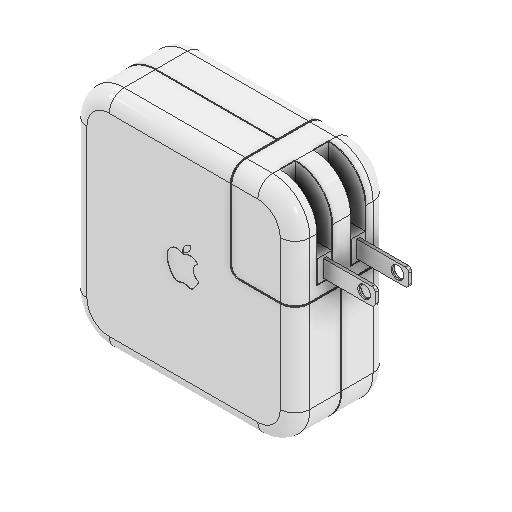
# Autodesk Inventor part: iPod Power Adapter
Saved by Autodesk Inventor 2026.2 (Build 302298000, 298)
## iProperties
Created: 2025-12-23
Part Number: iPod Power Adapter
Material: Generic
Document SubType Name: Modeling
Designer: andyeske
Density: 1 g/cm^3
Appearance: Default
Author: andyeske
Autodesk Inventor part; units mm, degrees
ref_plane "YZ Plane" through (0, 0, 0) normal (1, 0, 0) x (0, 1, 0)
ref_plane "XZ Plane" through (0, 0, 0) normal (0, 1, 0) x (-1, 0, 0)
ref_plane "XY Plane" through (0, 0, 0) normal (0, 0, 1) x (1, 0, 0)
sketch "Sketch1" plane through (0, 0, 0) normal (0, 0, 1) x (1, 0, 0)
  line L0 (-150, -150) -> (150, -150)
  line L1 (150, -150) -> (150, 150)
  line L2 (150, 150) -> (-150, 150)
  line L3 (-150, 150) -> (-150, -150)
  line L4 (-150, -150) -> (150, 150) construction
  line L5 (150, -150) -> (-150, 150) construction
  point P0 (0, 0)
  dimension "d0" = 300
  constraints: 12 end point, 2 midpoint, 2 parallel, 2 perpendicular, 1 horizontal
  measures "d0" distance of L1.end L2.end
extrude "Extrusion1" add sketch "Sketch1" along normal blind 125
fillet "Fillet1" radius 50 4 edges at (150, 150, 62.5) (-150, 150, 62.5) (150, -150, 62.5) (-150, -150, 62.5)
fillet "Fillet2" radius 20 16 edges at (0, 150, 125) (0, 150, 0) (-135.3553, 135.3553, 125) (-150, 0, 125) (-135.3553, -135.3553, 125) (0, -150, 125) (135.3553, -135.3553, 125) (150, 0, 125) (135.3553, 135.3553, 125) (-135.3553, 135.3553, 0) (-150, 0, 0) (-135.3553, -135.3553, 0) (0, -150, 0) (135.3553, -135.3553, 0) (150, 0, 0) (135.3553, 135.3553, 0)
sketch "Sketch2" plane through (0, 0, 125) normal (0, 0, 1) x (1, 0, 0)
  line L0 (100, 150) -> (-100, 150) projected
  line L1 (150, -100) -> (150, 100) projected
  line L2 (65, 150) -> (150, 150) construction
  line L3 (150, 150) -> (150, 25) construction
  line L4 (150, 25) -> (65, 25)
  line L5 (65, 25) -> (65, 150)
  line L6 (63, 150) -> (63, 23)
  line L7 (63, 23) -> (150, 23)
  line L8 (63, 150) -> (65, 150)
  point P0 (0, 0)
  dimension "d5" = 85
  dimension "d6" = 125
  dimension "d7" = 2
  dimension "d8" = 2
  constraints: 14 end point, 4 point on line, 2 parallel, 2 perpendicular, 1 collinear, 1 horizontal, 1 vertical
  measures "d5" distance of L3.end L4.end
  measures "d6" distance of L4.end L2.start
  measures "d7" distance between parallel lines of L5 L6
  measures "d8" distance between parallel lines of L7 L4
extrude "Extrusion2" cut sketch "Sketch2" against normal blind 1
sketch "Sketch3" plane through (-100, 150, 20) normal (0, 1, 0) x (1, 0, 0)
  line L0 (163, -104) -> (165, -104) projected
  line L1 (163, -104) -> (163, 0)
  line L2 (0, 0) -> (200, 0) projected
  line L3 (165, -104) -> (165, 0)
  line L4 (163, 0) -> (165, 0)
  point P0 (100, 20)
  constraints: 6 end point, 2 perpendicular, 2 point on line, 1 collinear
extrude "Extrusion3" cut sketch "Sketch3" against normal blind 1
sketch "Sketch4" plane through (150, -100, 20) normal (1, 0, 0) x (0, 0, -1)
  line L0 (-104, 125) -> (-104, 123) projected
  line L1 (-104, 125) -> (0, 125)
  line L2 (0, 200) -> (0, 0) projected
  line L3 (-104, 123) -> (0, 123)
  line L4 (0, 125) -> (0, 123)
  point P0 (20, 100)
  constraints: 6 end point, 2 point on line, 1 collinear, 1 horizontal, 1 perpendicular
extrude "Extrusion4" cut sketch "Sketch4" against normal blind 1
sketch "Sketch5" plane through (63, 23, 125) normal (1, 0, 0) x (0, 0, -1)
  arc A0 (20, 127) -> (0, 107) centre (20, 107) ccw projected
  arc A1 (20, 126) -> (1, 107) centre (20, 107) ccw
  line L0 (0, 107) -> (1, 107)
  line L1 (1, 0) -> (1, 113.245) projected
  line L2 (20, 126) -> (20, 127)
  point P0 (125, -23)
  dimension "d15" = 19
  constraints: 4 end point, 3 point on circle, 1 centre point, 1 point on line
  measures "d15" radius of A1
extrude "Extrusion5" cut sketch "Sketch5" along normal blind 2 contours L2 A1 L1 A0
sketch "Sketch6" plane through (63, 23, 125) normal (0, 1, 0) x (1, 0, 0)
  arc A0 (67, 0) -> (87, 20) centre (67, 20) ccw projected
  arc A1 (67, 1) -> (86, 20) centre (67, 20) ccw
  line L0 (86, 20) -> (87, 20)
  line L1 (86, 105) -> (86, 13.755) projected
  line L2 (73.245, 1) -> (0, 1) projected
  arc A2 (67, 0) -> (73.245, 1) centre (67, 20) ccw projected
  line L3 (67, 1) -> (67, 0)
  point P0 (-63, 125)
  dimension "d18" = 1
  constraints: 4 end point, 3 point on circle, 1 centre point, 1 perpendicular, 1 point on line
  measures "d18" radial gap between concentric circles of A0 A1
extrude "Extrusion6" cut sketch "Sketch6" along normal blind 2
sketch "Sketch7" plane through (0, 0, 0) normal (0, 0, -1) x (-1, 0, 0)
  line L0 (-63, 23) -> (-63, 130) projected
  line L1 (-130, 23) -> (-63, 23) projected
  line L2 (-65, 25) -> (-130, 25) projected
  line L3 (-65, 130) -> (-65, 25) projected
  line L4 (-65, 130) -> (-63, 130)
  line L5 (-130, 25) -> (-130, 23)
  point P0 (0, 0)
  constraints: 4 end point, 2 perpendicular
extrude "Extrusion7" cut sketch "Sketch7" against normal blind 1
sketch "Sketch8" plane through (63, 23, 125) normal (1, 0, 0) x (0, 0, -1)
  arc A0 (125, 107) -> (105, 127) centre (105, 107) ccw projected
  arc A1 (124, 107) -> (105, 126) centre (105, 107) ccw
  line L0 (105, 126) -> (105, 127)
  line L1 (125, 107) -> (124, 107) projected
  line L2 (124, 107) -> (125, 107)
  point P0 (125, -23)
  dimension "d23" = 1
  constraints: 4 end point, 2 point on circle, 1 centre point, 1 horizontal, 1 vertical
  measures "d23" radial gap between concentric circles of A0 A1
extrude "Extrusion8" cut sketch "Sketch8" along normal blind 2
sketch "Sketch9" plane through (63, 23, 125) normal (0, 1, 0) x (1, 0, 0)
  arc A0 (87, 105) -> (67, 125) centre (67, 105) ccw projected
  arc A1 (86, 105) -> (67, 124) centre (67, 105) ccw
  line L0 (67, 125) -> (67, 124) projected
  line L1 (67, 124) -> (67, 125)
  line L2 (86, 105) -> (87, 105)
  point P0 (-63, 125)
  dimension "d26" = 1
  constraints: 4 end point, 2 point on circle, 1 centre point, 1 horizontal, 1 vertical
  measures "d26" radial gap between concentric circles of A0 A1
extrude "Extrusion9" cut sketch "Sketch9" along normal blind 2
sketch "Sketch10" plane through (0, 0, 125) normal (0, 0, 1) x (1, 0, 0)
  line L0 (65, 25) -> (65, 130) projected
  line L1 (130, 25) -> (65, 25) projected
  arc A0 (65, 35) -> (75, 25) centre (75, 35) ccw
  line L2 (65, 35) -> (65, 25)
  point P0 (0, 0)
  dimension "d29" = 10
  constraints: 3 tangent, 2 end point, 2 point on circle, 2 point on line, 1 centre point, 1 collinear
  measures "d29" radius of A0
extrude "Extrusion10" cut sketch "Sketch10" against normal blind 1
sketch "Sketch11" plane through (0, 0, 125) normal (0, 0, 1) x (1, 0, 0)
  line L0 (63, 23) -> (63, 130) projected
  line L1 (63, 23) -> (130, 23) projected
  arc A0 (63, 35) -> (75, 23) centre (75, 35) ccw
  arc A1 (65, 35) -> (75, 25) centre (75, 35) ccw projected
  line L2 (63, 35) -> (63, 23)
  point P0 (0, 0)
  constraints: 3 tangent, 2 end point, 2 point on circle, 2 point on line, 1 centre point, 1 collinear, 1 concentric
extrude "Extrusion11" add sketch "Sketch11" against normal blind 1
sketch "Sketch12" plane through (0, 0, 0) normal (0, 0, -1) x (-1, 0, 0)
  arc A0 (-75, 25) -> (-65, 35) centre (-75, 35) ccw projected
  line L0 (-130, 25) -> (-65, 25) projected
  line L1 (-75, 25) -> (-65, 25)
  line L2 (-65, 25) -> (-65, 35)
  point P0 (0, 0)
  constraints: 4 end point, 1 horizontal, 1 perpendicular
extrude "Extrusion12" cut sketch "Sketch12" against normal blind 1
sketch "Sketch13" plane through (0, 0, 0) normal (0, 0, -1) x (-1, 0, 0)
  arc A0 (-75, 23) -> (-63, 35) centre (-75, 35) ccw projected
  line L0 (-63, 130) -> (-63, 23) projected
  line L1 (-63, 35) -> (-63, 23)
  line L2 (-63, 23) -> (-75, 23)
  point P0 (0, 0)
  constraints: 4 end point, 1 perpendicular, 1 tangent, 1 vertical
extrude "Extrusion13" add sketch "Sketch13" against normal blind 1
sketch "Sketch14" plane through (-100, 150, 105) normal (0, 1, 0) x (1, 0, 0)
  line L0 (163, 0) -> (163, 85) construction
  line L1 (163, 42.5) -> (0, 42.5) construction
  line L2 (0, 85) -> (0, 0) construction
  line L3 (0, 42) -> (163, 42)
  line L4 (163, 42) -> (163, 43)
  line L5 (163, 43) -> (0, 43)
  line L6 (0, 43) -> (0, 42)
  line L7 (0, 42) -> (163, 43) construction
  line L8 (163, 42) -> (0, 43) construction
  point P0 (100, 105)
  point P1 (81.5, 42.5)
  dimension "d38" = 1
  constraints: 14 end point, 5 midpoint, 2 parallel, 1 horizontal, 1 perpendicular, 1 point on line
  measures "d38" distance between parallel lines of L3 L5
extrude "Extrusion14" cut sketch "Sketch14" against normal blind 0.5
sketch "Sketch15" plane through (-150, -100, 20) normal (-1, 0, 0) x (0, 0, 1)
  line L0 (0, 200) -> (85, 200) construction
  line L1 (42.5, 200) -> (42.5, 0) construction
  line L2 (85, 0) -> (0, 0) construction
  line L3 (43, 0) -> (42, 0)
  line L4 (42, 0) -> (42, 200)
  line L5 (42, 200) -> (43, 200)
  line L6 (43, 200) -> (43, 0)
  line L7 (43, 0) -> (42, 200) construction
  line L8 (42, 0) -> (43, 200) construction
  point P0 (-20, 100)
  point P1 (42.5, 100)
  dimension "d41" = 1
  constraints: 14 end point, 5 midpoint, 2 parallel, 1 horizontal, 1 perpendicular, 1 point on line
  measures "d41" distance between parallel lines of L6 L4
extrude "Extrusion15" cut sketch "Sketch15" against normal blind 0.5
sketch "Sketch16" plane through (-100, -150, 20) normal (0, -1, 0) x (1, 0, 0)
  line L0 (200, 85) -> (200, 0) construction
  line L1 (200, 42.5) -> (0, 42.5) construction
  line L2 (0, 0) -> (0, 85) construction
  line L3 (200, 43) -> (0, 43)
  line L4 (0, 43) -> (0, 42)
  line L5 (0, 42) -> (200, 42)
  line L6 (200, 42) -> (200, 43)
  line L7 (200, 43) -> (0, 42) construction
  line L8 (0, 43) -> (200, 42) construction
  point P0 (100, -20)
  point P1 (100, 42.5)
  dimension "d44" = 1
  constraints: 14 end point, 5 midpoint, 2 parallel, 1 horizontal, 1 perpendicular, 1 point on line
  measures "d44" distance between parallel lines of L3 L5
extrude "Extrusion16" cut sketch "Sketch16" against normal blind 0.5
sketch "Sketch17" plane through (150, -100, 105) normal (1, 0, 0) x (0, 0, -1)
  line L0 (42.5, 0) -> (38.8069, 200) construction
  line L1 (42.5, 0) -> (42.5, 123) construction
  line L2 (85, 123) -> (0, 123) construction
  line L3 (0, 0) -> (42, 0) projected
  line L4 (43, 123) -> (42, 123)
  line L5 (42, 123) -> (42, 0)
  line L6 (42, 0) -> (43, 0)
  line L7 (43, 0) -> (43, 123)
  line L8 (43, 123) -> (42, 0) construction
  line L9 (42, 123) -> (43, 0) construction
  line L10 (85, 123) -> (85, 0) construction
  line L11 (85, 61.5) -> (42.5, 61.5) construction
  point P0 (105, 100)
  dimension "d47" = 1
  dimension "d53" = 42.5
  constraints: 18 end point, 5 midpoint, 2 parallel, 2 perpendicular, 1 horizontal, 1 point on line, 1 vertical
  measures "d47" distance between parallel lines of L5 L7
  measures "d53" distance of L11.start L11.end
extrude "Extrusion17" cut sketch "Sketch17" against normal blind 0.5
sketch "Sketch18" plane through (-150, -100, 63) normal (0, 0, -1) x (-1, 0, 0)
  arc A0 (0, 200) -> (-50, 250) centre (-50, 200) ccw projected
  arc A1 (-50, -50) -> (0, 0) centre (-50, 0) ccw projected
  arc A2 (-300, 0) -> (-250, -50) centre (-250, 0) ccw projected
  arc A3 (-299.5, 0) -> (-250, -49.5) centre (-250, 0) ccw
  arc A4 (-50, -49.5) -> (-0.5, 0) centre (-50, 0) ccw
  arc A5 (-0.5, 200) -> (-50, 249.5) centre (-50, 200) ccw
  line L0 (-0.5, 200) -> (0, 200)
  line L1 (-50, 250) -> (-50, 249.5) projected
  line L2 (0, 0) -> (-0.5, 0) projected
  line L3 (-50, -50) -> (-50, -49.5) projected
  line L4 (-250, -50) -> (-250, -49.5) projected
  line L5 (-300, 0) -> (-299.5, 0) projected
  point P0 (-150, 100)
  dimension "d50" = 0.5
  dimension "d51" = 0.5
  dimension "d52" = 0.5
  constraints: 6 point on circle, 5 point on line, 3 centre point, 2 end point, 1 horizontal
  measures "d50" radial gap between concentric circles of A2 A3
  measures "d51" radial gap between concentric circles of A1 A4
  measures "d52" radial gap between concentric circles of A0 A5
extrude "Extrusion18" cut sketch "Sketch18" along normal blind 1
sketch "Sketch19" plane through (0, 0, 125) normal (0, 0, 1) x (1, 0, 0)
  line L0 (-25.8842, 32.2382) -> (24.1158, 32.2382) construction
  line L1 (24.1158, 32.2382) -> (24.1158, -21.8992) construction
  line L2 (24.1158, -21.8992) -> (-25.8842, -21.8992) construction
  line L3 (-25.8842, -21.8992) -> (-25.8842, 32.2382) construction
  spline S0 degree 4 poles (-0.6067, 15.9177) (2.7295, 16.3934) (4.6914, 19.5945) (14.5472, 18.5482) (17.2027, 15.3244) (18.6949, 13.3249) knots 0 0 0 0 0 0.505773 1 1 1 1 1
  spline S1 degree 4 poles (18.6949, 13.3249) (17.4559, 12.3952) (13.095, 9.7666) (11.88, 0.5556) (16.3487, -4.4756) (18.9422, -6.1803) (20.1095, -6.4916) knots 0 0 0 0 0 0.441121 0.625892 1 1 1 1 1
  spline S2 degree 4 poles (20.1095, -6.4916) (19.0498, -10.0156) (18.7751, -10.1929) (13.7906, -17.7207) (11.0782, -19.5298) (7.8639, -20.2186) (5.3082, -19.0784) (0.7675, -17.5229) (-2.0147, -18.0206) (-6.006, -19.5989) (-9.1544, -20.4858) (-13.1462, -18.1919) (-14.7306, -15.8813) (-18.6351, -10.7741) (-19.3629, -8.5442) (-22.322, -1.3736) (-21.8645, 4.1613) (-21.7165, 10.1898) (-17.7625, 15.2877) (-10.9125, 18.9157) (-7.1098, 18.7842) (-2.3164, 15.9818) (-0.6067, 15.9177) knots 0 0 0 0 0 0.113024 0.15496 0.194895 0.233325 0.273058 0.315021 0.3576 0.399129 0.440951 0.48455 0.528381 0.575776 0.626758 0.678413 0.73359 0.787538 0.838503 0.887902 1 1 1 1 1
  arc A0 (9.5273, 30.1366) -> (-0.8842, 18.2584) centre (10.1214, 19.1138) ccw
  arc A1 (-0.8842, 18.2584) -> (9.5273, 30.1366) centre (-1.5571, 29.3502) ccw
  point P0 (0, 0)
  point P1 (3.3905, 17.2501)
  point P2 (7.0996, 18.2584)
  point P3 (12.4291, 17.7902)
  point P4 (16.3182, 15.9177)
  point P5 (16.3182, 11.4164)
  point P6 (13.5094, 6.771)
  point P7 (13.5609, 0.7964)
  point P8 (15.849, -3.3903)
  point P9 (18.4293, -5.6785)
  point P10 (18.6949, -10.1752)
  point P11 (16.3182, -13.7425)
  point P12 (12.7147, -18.1632)
  point P13 (10.6394, -19.4677)
  point P14 (8.1689, -19.863)
  point P15 (5.3425, -19.1514)
  point P16 (1.0358, -17.9357)
  point P17 (-2.1974, -18.2296)
  point P18 (-5.9382, -19.4854)
  point P19 (-9.2248, -19.8595)
  point P20 (-12.5651, -18.2562)
  point P21 (-14.8899, -15.7181)
  point P22 (-17.9783, -11.3749)
  point P23 (-19.5146, -8.2718)
  point P24 (-21.5699, -1.9875)
  point P25 (-21.9056, 4.2826)
  point P26 (-20.8879, 10.1017)
  point P27 (-17.1455, 15.106)
  point P28 (-12.3285, 17.7902)
  point P29 (-8.4965, 18.2584)
  point P30 (-4.0648, 16.9966)
  dimension "d59" = 50
  constraints: 4 point on circle, 2 centre point, 38 other
  measures "d59" distance of L1.end L2.end
extrude "Extrusion19" cut sketch "Sketch19" against normal blind 0.5
sketch "Sketch20" plane through (0, 0, 0) normal (0, 0, -1) x (-1, 0, 0)
  line L0 (-26.5297, 33.619) -> (23.4703, 33.619) construction
  line L1 (23.4703, 33.619) -> (23.4703, -20.5184) construction
  line L2 (23.4703, -20.5184) -> (-26.5297, -20.5184) construction
  line L3 (-26.5297, -20.5184) -> (-26.5297, 33.619) construction
  spline S0 degree 4 poles (-1.2521, 17.2985) (2.084, 17.7743) (4.046, 20.9753) (13.9017, 19.929) (16.5573, 16.7052) (18.0494, 14.7058) knots 0 0 0 0 0 0.505773 1 1 1 1 1
  spline S1 degree 4 poles (18.0494, 14.7058) (16.8105, 13.776) (12.4496, 11.1474) (11.2345, 1.9364) (15.7032, -3.0948) (18.2967, -4.7995) (19.464, -5.1108) knots 0 0 0 0 0 0.441121 0.625892 1 1 1 1 1
  spline S2 degree 4 poles (19.464, -5.1108) (18.4043, -8.6348) (18.1296, -8.8121) (13.1451, -16.3399) (10.4327, -18.149) (7.2184, -18.8378) (4.6628, -17.6976) (0.122, -16.1421) (-2.6601, -16.6398) (-6.6515, -18.218) (-9.7999, -19.1049) (-13.7916, -16.8111) (-15.3761, -14.5005) (-19.2806, -9.3932) (-20.0084, -7.1634) (-22.9675, 0.0072) (-22.51, 5.5421) (-22.362, 11.5706) (-18.4079, 16.6686) (-11.558, 20.2965) (-7.7553, 20.165) (-2.9619, 17.3626) (-1.2521, 17.2985) knots 0 0 0 0 0 0.113024 0.15496 0.194895 0.233325 0.273058 0.315021 0.3576 0.399129 0.440951 0.48455 0.528381 0.575776 0.626758 0.678413 0.73359 0.787538 0.838503 0.887902 1 1 1 1 1
  arc A0 (8.8818, 31.5175) -> (-1.5297, 19.6392) centre (9.476, 20.4946) ccw
  arc A1 (-1.5297, 19.6392) -> (8.8818, 31.5175) centre (-2.2026, 30.731) ccw
  point P0 (0, 0)
  point P1 (-0.6455, 1.3808)
  point P2 (2.745, 18.6309)
  point P3 (6.4541, 19.6392)
  point P4 (11.7836, 19.171)
  point P5 (15.6728, 17.2985)
  point P6 (15.6727, 12.7972)
  point P7 (12.8639, 8.1519)
  point P8 (12.9155, 2.1773)
  point P9 (15.2036, -2.0095)
  point P10 (17.7838, -4.2977)
  point P11 (18.0494, -8.7944)
  point P12 (15.6727, -12.3617)
  point P13 (12.0692, -16.7824)
  point P14 (9.9939, -18.0868)
  point P15 (7.5234, -18.4821)
  point P16 (4.6971, -17.7706)
  point P17 (0.3903, -16.5549)
  point P18 (-2.8429, -16.8488)
  point P19 (-6.5837, -18.1046)
  point P20 (-9.8703, -18.4787)
  point P21 (-13.2105, -16.8754)
  point P22 (-15.5354, -14.3372)
  point P23 (-18.6238, -9.994)
  point P24 (-20.1601, -6.891)
  point P25 (-22.2154, -0.6066)
  point P26 (-22.551, 5.6634)
  point P27 (-21.5333, 11.4825)
  point P28 (-17.791, 16.4868)
  point P29 (-12.974, 19.1711)
  point P30 (-9.142, 19.6392)
  point P31 (-4.7103, 18.3775)
  dimension "d79" = 50
  constraints: 4 point on circle, 2 centre point, 37 other
  measures "d79" distance of L1.end L3.start
extrude "Extrusion20" cut sketch "Sketch20" against normal blind 0.5
sketch "Sketch21" plane through (-150, -100, 20) normal (-1, 0, 0) x (0, 0, 1)
  line L0 (0, 0) -> (0, 200) construction
  line L1 (0, 100) -> (85, 100) construction
  line L2 (85, 0) -> (85, 123) construction
  circle A0 centre (42.5, 100) radius 30
  circle A1 centre (42.5, 100) radius 31
  point P0 (-20, 100)
  dimension "d85" = 60
  dimension "d86" = 1
  constraints: 2 centre point, 2 end point, 2 midpoint, 1 horizontal, 1 point on line
  measures "d85" diameter of A0
  measures "d86" radial gap between concentric circles of A0 A1
extrude "Extrusion21" cut sketch "Sketch21" against normal up to surface (0.5 mm away)
sketch "Sketch22" plane through (-150, 0, 62.5) normal (-1, 0, 0) x (0, 0, 1)
  point P0 (-62.5, 0)
extrude "Extrusion22" add sketch "Sketch21" against normal up to surface (0.5 mm away) contours A0
sketch "Sketch23" plane through (-150, 0, 62.5) normal (-1, 0, 0) x (0, 0, 1)
  circle A0 centre (0, 0) radius 30 construction
  line L0 (0, 30) -> (0, -30) construction
  line L1 (0.5, -100) -> (0.5, 23) construction
  line L2 (0, 0) -> (42.5, 0) construction
  line L3 (42.5, 100) -> (42.5, -100) construction
  line L4 (-10, -25) -> (10, -25)
  line L5 (10, -25) -> (10, 25)
  line L6 (10, 25) -> (-10, 25)
  line L7 (-10, 25) -> (-10, -25)
  line L8 (-10, -25) -> (10, 25) construction
  line L9 (10, -25) -> (-10, 25) construction
  point P0 (-62.5, 0)
  dimension "d91" = 42.5
  dimension "d92" = 20
  dimension "d93" = 50
  constraints: 16 end point, 4 midpoint, 3 parallel, 2 point on circle, 1 horizontal, 1 perpendicular
  measures "d91" distance of L2.start L2.end
  measures "d92" distance of L5.end L6.end
  measures "d93" distance of L4.end L5.end
extrude "Extrusion23" cut sketch "Sketch23" against normal blind 50
chamfer "Chamfer1" distance 0.5 angle 45 4 edges at (-150, 25, 62.5) (-150, 0, 52.5) (-150, 0, 72.5) (-150, -25, 62.5)
sketch "Sketch24" plane through (100, 150, 105) normal (0, 1, 0) x (1, 0, 0)
  line L0 (50, 0) -> (50, 85) projected
  line L1 (0, 43) -> (0, 85) projected
  line L2 (50, 75) -> (0, 75)
  line L3 (0, 75) -> (0, 55)
  line L4 (0, 55) -> (50, 55)
  line L5 (50, 55) -> (50, 75)
  line L6 (50, 30) -> (0, 30)
  line L7 (0, 30) -> (0, 10)
  line L8 (0, 10) -> (50, 10)
  line L9 (50, 10) -> (50, 30)
  line L10 (50, 85) -> (0, 85) projected
  line L11 (0, 0) -> (50, 0) projected
  point P0 (-100, 105)
  point P1 (0, 75)
  point P2 (50, 10)
  point P3 (50, 30)
  dimension "d99" = 10
  dimension "d100" = 10
  dimension "d101" = 20
  dimension "d102" = 20
  constraints: 16 end point, 4 parallel, 4 point on line, 2 horizontal, 2 perpendicular
  measures "d99" distance between parallel lines of L2 L10
  measures "d100" distance between parallel lines of L11 L8
  measures "d101" distance between parallel lines of L4 L2
  measures "d102" distance between parallel lines of L8 L6
extrude "Extrusion24" cut sketch "Sketch24" against normal blind 110 contours L8 L7 L6 L0 | L4 L1 L2 L0
fillet "Fillet3" radius 0.5 12 edges at (100, 150, 85) (150, 70, 75) (135.3553, 135.3553, 75) (150, 70, 95) (135.3553, 135.3553, 95) (100, 150, 40) (150, 70, 50) (135.3553, 135.3553, 50) (150, 70, 30) (135.3553, 135.3553, 30) (150, 40, 40) (150, 40, 85)
sketch "Sketch25" plane through (100, 40, 30) normal (0, 0, 1) x (1, 0, 0)
  line L0 (-1.2951, 0.5) -> (50, 0.5)
  line L1 (50, 0.5) -> (50, 30.5)
  line L2 (50, 30.5) -> (-1.2951, 30.5)
  line L3 (-1.2951, 30.5) -> (-1.2951, 0.5)
  line L4 (50, -0.5) -> (50, 60) projected
  line L5 (0, 0) -> (49.5, 0) projected
  point P0 (-100, -40)
  dimension "d106" = 0.5
  dimension "d113" = 30
  constraints: 8 end point, 2 parallel, 1 collinear, 1 horizontal, 1 perpendicular
  measures "d106" distance between parallel lines of L5 L0
  measures "d113" distance between parallel lines of L0 L2
extrude "Extrusion25" add sketch "Sketch25" along normal up to surface (20 mm away)
sketch "Sketch26" plane through (150, 40.5, 30) normal (1, 0, 0) x (0, 0, -1)
  line L0 (-20, 30) -> (0, 30) projected
  line L1 (0, 0) -> (-20, 0) projected
  line L2 (-20, 30) -> (-19.5, 30)
  line L3 (-19.5, 30) -> (-19.5, 0)
  line L4 (-19.5, 0) -> (-20, 0)
  line L5 (-20, 0) -> (-20, 30)
  line L6 (0, 30) -> (-20, 30) projected
  line L7 (0, 30) -> (-0.5, 30)
  line L8 (-0.5, 30) -> (-0.5, 0)
  line L9 (-0.5, 0) -> (0, 0)
  line L10 (0, 0) -> (0, 30)
  point P0 (30, -40.5)
  point P1 (0, 0)
  point P2 (-20, 0)
  dimension "d109" = 0.5
  dimension "d110" = 0.5
  constraints: 16 end point, 4 parallel, 2 horizontal, 2 perpendicular, 2 point on line
  measures "d109" distance between parallel lines of L10 L8
  measures "d110" distance between parallel lines of L5 L3
extrude "Extrusion26" cut sketch "Sketch26" against normal up to surface (50 mm away) contours L0 L3 L1 L5 | L0 L10 L1 L8
sketch "Sketch27" plane through (100, 40, 75) normal (0, 0, 1) x (1, 0, 0)
  line L0 (50, 30.5) -> (-1.2951, 30.5) projected
  line L1 (0, 0.5) -> (50, 0.5) projected
  line L2 (0, 109.5) -> (0, 0) projected
  line L3 (0, 30.5) -> (0, 0.5)
  line L4 (50, 30.5) -> (50, 0.5)
  point P0 (-100, -40)
  constraints: 4 end point, 2 point on line, 1 perpendicular, 1 vertical
extrude "Extrusion27" add sketch "Sketch27" along normal up to surface (20 mm away)
sketch "Sketch28" plane through (150, 40.5, 75) normal (1, 0, 0) x (0, 0, -1)
  line L0 (-20, 30) -> (0, 30) projected
  line L1 (0, 0) -> (-20, 0) projected
  line L2 (-20, 30) -> (-19.5, 30)
  line L3 (-19.5, 30) -> (-19.5, 0)
  line L4 (-19.5, 0) -> (-20, 0)
  line L5 (-20, 0) -> (-20, 30)
  line L6 (0, 30) -> (-0.5, 30)
  line L7 (-0.5, 30) -> (-0.5, 0)
  line L8 (-0.5, 0) -> (0, 0)
  line L9 (0, 0) -> (0, 30)
  point P0 (75, -40.5)
  point P1 (-0.5, 30)
  point P2 (-19.5, 30)
  dimension "d116" = 0.5
  dimension "d117" = 0.5
  constraints: 16 end point, 4 parallel, 2 horizontal, 2 perpendicular, 2 point on line
  measures "d116" distance between parallel lines of L5 L3
  measures "d117" distance between parallel lines of L9 L7
extrude "Extrusion28" cut sketch "Sketch28" against normal up to surface (50 mm away) contours L0 L3 L1 L5 | L0 L9 L1 L7
sketch "Sketch29" plane through (150, 40.5, 75.5) normal (1, 0, 0) x (0, 0, -1)
  line L0 (45, 30) -> (26, 30) construction
  line L1 (35.5, 30) -> (35.5, 0) construction
  line L2 (45, 0) -> (26, 0) construction
  line L3 (0, 30) -> (-19, 30) construction
  line L4 (-9.5, 30) -> (-9.5, 0) construction
  line L5 (0, 0) -> (-19, 0) construction
  line L6 (33.5, 3.5) -> (37.5, 3.5)
  line L7 (37.5, 3.5) -> (37.5, 26.5)
  line L8 (37.5, 26.5) -> (33.5, 26.5)
  line L9 (33.5, 26.5) -> (33.5, 3.5)
  line L10 (33.5, 3.5) -> (37.5, 26.5) construction
  line L11 (37.5, 3.5) -> (33.5, 26.5) construction
  line L12 (-11.5, 3.5) -> (-7.5, 3.5)
  line L13 (-7.5, 3.5) -> (-7.5, 26.5)
  line L14 (-7.5, 26.5) -> (-11.5, 26.5)
  line L15 (-11.5, 26.5) -> (-11.5, 3.5)
  line L16 (-11.5, 3.5) -> (-7.5, 26.5) construction
  line L17 (-7.5, 3.5) -> (-11.5, 26.5) construction
  point P0 (75.5, -40.5)
  point P1 (35.5, 15)
  point P2 (-9.5, 15)
  dimension "d120" = 23
  dimension "d121" = 4
  constraints: 28 end point, 10 midpoint, 4 parallel, 2 horizontal, 2 perpendicular, 1 collinear, 1 point on line
  measures "d120" distance of L12.end L13.end
  measures "d121" distance of L13.end L14.end
extrude "Extrusion29" add sketch "Sketch29" along normal blind 70
fillet "Fillet4" radius 5 4 edges at (220, 67, 85) (220, 67, 40) (220, 44, 40) (220, 44, 85)
sketch "Sketch30" plane through (150, 44, 87) normal (0, 0, 1) x (1, 0, 0)
  line L0 (70, 18) -> (70, 5) construction
  line L1 (70, 11.5) -> (55, 11.5) construction
  circle A0 centre (55, 11.5) radius 7.5
  point P0 (-150, -44)
  dimension "d125" = 15
  dimension "d126" = 15
  constraints: 2 end point, 1 centre point, 1 coincident, 1 horizontal, 1 midpoint
  measures "d125" diameter of A0
  measures "d126" distance of L1.start L1.end
extrude "Extrusion30" cut sketch "Sketch30" against normal through all
fillet "Fillet5" radius 1 4 edges at (197.5, 55.5, 87) (197.5, 55.5, 42) (197.5, 55.5, 83) (197.5, 55.5, 38)
body "Solid1"
